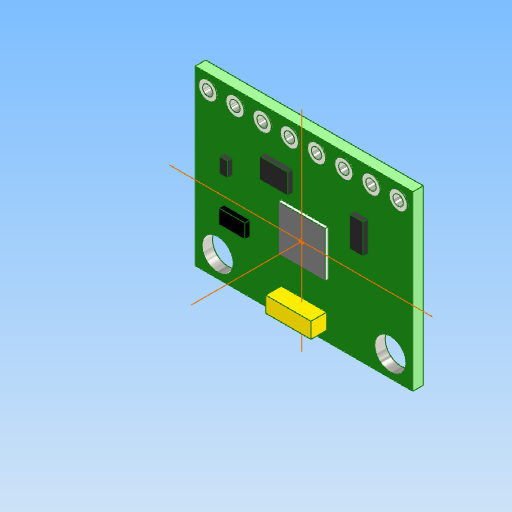
# Autodesk Inventor part: MPU6050
Saved by Autodesk Inventor 2021.2 (Build 252289000, 289)
## iProperties
Created: 2025-04-06
Part Number: MPU6050
Material: Типовые
Document SubType Name: Modeling
Designer: barko
Density: 8.66084 g/cm^3
Appearance: По умолчанию
Mass: 3 g
Surface Area: 8.08705 cm^2
Volume: 0.346387 cm^3
Author: barko
Autodesk Inventor part; units mm, degrees
ref_plane "YZ Plane" through (0, 0, 0) normal (1, 0, 0) x (0, 1, 0)
ref_plane "XZ Plane" through (0, 0, 0) normal (0, 1, 0) x (-1, 0, 0)
ref_plane "XY Plane" through (0, 0, 0) normal (0, 0, 1) x (1, 0, 0)
sketch "Эскиз1" plane through (0, 0, 0) normal (0, 0, 1) x (1, 0, 0)
  line L0 (10.4, -8.25) -> (-10.4, -8.25)
  line L1 (-10.4, -8.25) -> (-10.4, 8.25)
  line L2 (-10.4, 8.25) -> (10.4, 8.25)
  line L3 (10.4, 8.25) -> (10.4, -8.25)
  line L4 (10.4, -8.25) -> (-10.4, 8.25) construction
  line L5 (-10.4, -8.25) -> (10.4, 8.25) construction
  circle A0 centre (-8.25, -6.25) radius 1.5
  circle A1 centre (8.25, -6.25) radius 1.5
  circle A2 centre (-9.1, 6.95) radius 0.5
  circle A3 centre (-9.1, 6.95) radius 0.875
  line L6 (-10.4, 6.95) -> (10.4, 6.95) construction
  point P0 (0, 0)
  dimension "d0" = 20.8
  dimension "d1" = 16.5
  dimension "d2" = 3
  dimension "d3" = 3
  dimension "d4" = 13.5
  dimension "d5" = 0.5
  dimension "d8" = 2.15
  dimension "d9" = 2.15
  dimension "d10" = 1
  dimension "d11" = 1.75
  dimension "d12" = 1.3
  dimension "d13" = 1.3
  constraints: 14 end point, 4 centre point, 3 point on line, 2 midpoint, 2 parallel, 2 perpendicular, 1 coincident, 1 horizontal, 1 horizontal alignment
  measures "d0" distance of L1.end L2.end
  measures "d1" distance of L0.end L1.end
  measures "d2" diameter of A0
  measures "d3" diameter of A1
  measures "d5" distance edge to line of A0 L0
  measures "d8" distance from line of L3 A1.centre
  measures "d9" distance from line of A0.centre L1
  measures "d10" diameter of A2
  measures "d11" diameter of A3
  measures "d12" distance between parallel lines of L2 L6
  measures "d13" distance from line of A2.centre L1
extrude "Выдавливание1" add sketch "Эскиз1" along normal blind 1 contours L0 L1 L2 L3 | A2 | A3
extrude "Выдавливание2" cut sketch "Эскиз1" along normal blind 1.5 contours A2
extrude "Выдавливание3" add sketch "Эскиз1" along normal blind 0.1 from surface at 1 contours A3
pattern_linear "Прямоуг.массив1" count 8 spacing 2.6 along (1, 0, 0) of "Выдавливание3", "Выдавливание2"
sketch "Эскиз2" plane through (0, 0, 1) normal (0, 0, 1) x (1, 0, 0)
  line L0 (2.3179, -3.0275) -> (-2.1648, -3.0275)
  line L1 (-2.1648, -3.0275) -> (-2.1648, 1.3166)
  line L2 (-2.1648, 1.3166) -> (2.3179, 1.3166)
  line L3 (2.3179, 1.3166) -> (2.3179, -3.0275)
  line L4 (2.3179, -3.0275) -> (-2.1648, 1.3166) construction
  line L5 (-2.1648, -3.0275) -> (2.3179, 1.3166) construction
  line L6 (-2.1648, -5.8271) -> (2.1648, -5.8271)
  line L7 (2.1648, -5.8271) -> (2.1648, -7.3246)
  line L8 (2.1648, -7.3246) -> (-2.1648, -7.3246)
  line L9 (-2.1648, -7.3246) -> (-2.1648, -5.8271)
  line L10 (-2.1648, -5.8271) -> (2.1648, -7.3246) construction
  line L11 (2.1648, -5.8271) -> (-2.1648, -7.3246) construction
  line L12 (-7.6013, 2.4415) -> (-6.82, 2.4415)
  line L13 (-6.82, 2.4415) -> (-6.82, 1.0092)
  line L14 (-6.82, 1.0092) -> (-7.6013, 1.0092)
  line L15 (-7.6013, 1.0092) -> (-7.6013, 2.4415)
  line L16 (-7.6013, 2.4415) -> (-6.82, 1.0092) construction
  line L17 (-6.82, 2.4415) -> (-7.6013, 1.0092) construction
  line L18 (4.8419, 3.8739) -> (6.1364, 3.8739)
  line L19 (6.1364, 3.8739) -> (6.1364, 1.0092)
  line L20 (6.1364, 1.0092) -> (4.8419, 1.0092)
  line L21 (4.8419, 1.0092) -> (4.8419, 3.8739)
  line L22 (4.8419, 3.8739) -> (6.1364, 1.0092) construction
  line L23 (6.1364, 3.8739) -> (4.8419, 1.0092) construction
  line L24 (-3.7552, 4.3914) -> (-1.058, 4.3914)
  line L25 (-1.058, 4.3914) -> (-1.058, 2.4415)
  line L26 (-1.058, 2.4415) -> (-3.7552, 2.4415)
  line L27 (-3.7552, 2.4415) -> (-3.7552, 4.3914)
  line L28 (-3.7552, 4.3914) -> (-1.058, 2.4415) construction
  line L29 (-1.058, 4.3914) -> (-3.7552, 2.4415) construction
  line L30 (-7.6406, -1.8556) -> (-5.153, -1.8556)
  line L31 (-5.153, -1.8556) -> (-5.153, -3.2228)
  line L32 (-5.153, -3.2228) -> (-7.6406, -3.2228)
  line L33 (-7.6406, -3.2228) -> (-7.6406, -1.8556)
  line L34 (-7.6406, -1.8556) -> (-5.153, -3.2228) construction
  line L35 (-5.153, -1.8556) -> (-7.6406, -3.2228) construction
  point P0 (0, 0)
  point P1 (0.0765, -0.8555)
  point P2 (0, -6.5758)
  point P3 (-7.2106, 1.7253)
  point P4 (5.4892, 2.4415)
  point P5 (-2.4066, 3.4165)
  point P6 (-6.3968, -2.5392)
  constraints: 72 end point, 12 midpoint, 12 parallel, 6 horizontal, 6 perpendicular, 3 point on line
extrude "Выдавливание4" add sketch "Эскиз2" along normal blind 0.3 contours L0 L1 L2 L3
extrude "Выдавливание5" add sketch "Эскиз2" along normal blind 1.5 contours L6 L7 L8 L9
extrude "Выдавливание6" add sketch "Эскиз2" along normal blind 0.5 contours L12 L13 L14 L15 | L18 L19 L20 L21 | L24 L25 L26 L27 | L30 L31 L32 L33
sketch "Эскиз3" plane through (0, 0, 1.3) normal (0, 0, 1) x (1, 0, 0)
  line L0 (2.3179, 1.3166) -> (-2.1648, 1.3166) construction
  line L1 (-2.1648, 1.3166) -> (-2.1648, -3.0275) construction
  line L2 (-2.1648, -3.0275) -> (2.3179, -3.0275) construction
  line L3 (2.3179, -3.0275) -> (2.3179, 1.3166) construction
  point P0 (0, 0)
  point P1 (0.0765, -0.8555)
  point P2 (0.0765, 1.3166)
  point P3 (2.3179, -0.8555)
  constraints: 2 midpoint, 1 horizontal alignment, 1 vertical alignment
equation "\"d8\" = d9"
equation "\"d13\" = 0.0625 * d0"
equation "\"d22\" = 2 * d13"
